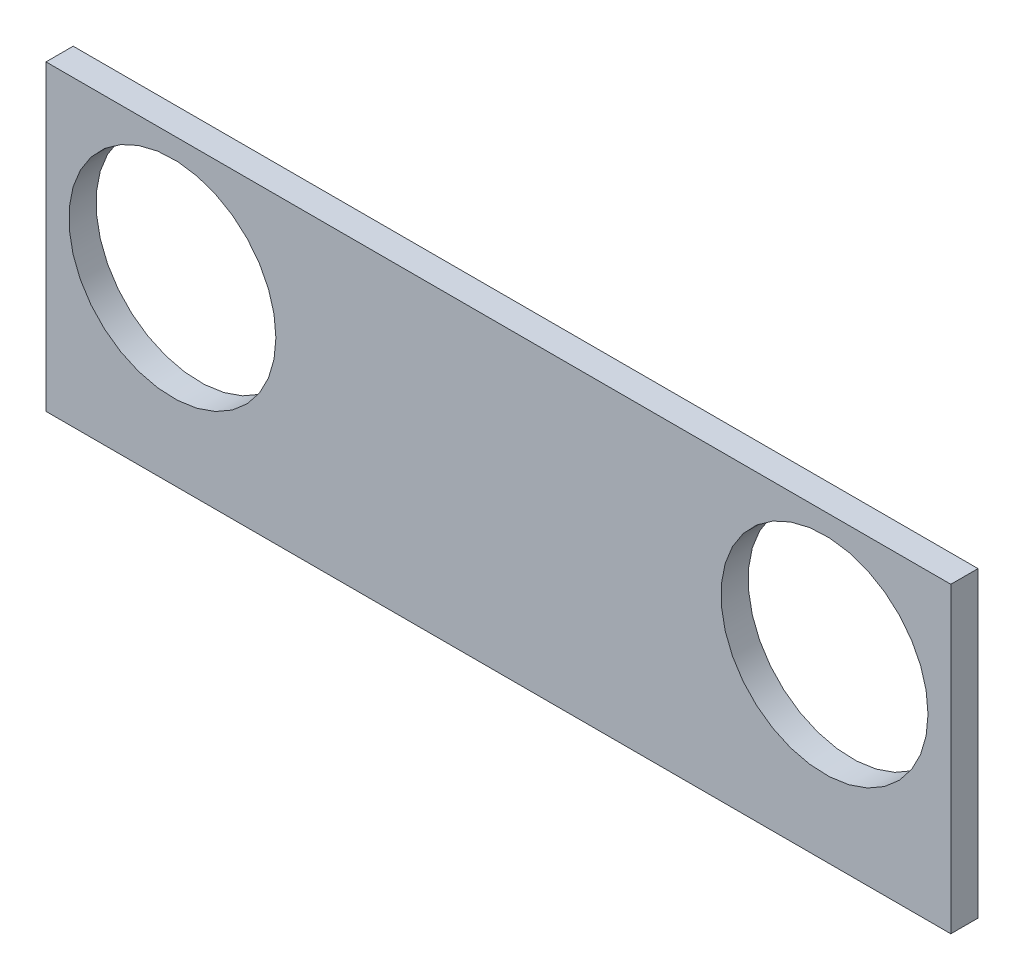
# Autodesk Inventor part: vaz
Saved by Autodesk Inventor 2019 (Build 230136000, 136)
## iProperties
Created: 2020-04-03
Part Number: vaz
Material: Generic
Document SubType Name: Modeling
Designer: laca
Density: 1 g/cm^3
Appearance: Default
Author: laca
Autodesk Inventor part; units mm, degrees
ref_plane "YZ Plane" through (0, 0, 0) normal (1, 0, 0) x (0, 1, 0)
ref_plane "XZ Plane" through (0, 0, 0) normal (0, 1, 0) x (-1, 0, 0)
ref_plane "XY Plane" through (0, 0, 0) normal (0, 0, 1) x (1, 0, 0)
sketch "Sketch1" plane through (0, 0, 0) normal (0, 0, 1) x (1, 0, 0)
  circle A0 centre (0, 0) radius 38.1
  circle A1 centre (240, 0) radius 38.1
  line L0 (-46.513, -65.7871) -> (286.4945, -65.7871)
  line L1 (286.4945, -65.7871) -> (286.4945, 45.6215)
  line L2 (286.4945, 45.6215) -> (-46.513, 45.6215)
  line L3 (-46.513, 45.6215) -> (-46.513, -65.7871)
  dimension "d0" = 76.2
  dimension "d1" = 76.2
  dimension "d2" = 240
  constraints: 8 end point, 2 centre point, 2 parallel, 1 coincident, 1 horizontal, 1 perpendicular
  measures "d0" diameter of A0
  measures "d1" diameter of A1
  measures "d2" distance of A1.centre point (0, 0)
extrude "Extrusion1" add sketch "Sketch1" along normal blind 10
body "Solid1"
